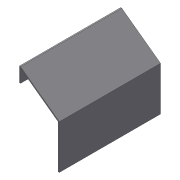
# Autodesk Inventor part: タイヤカバー
Saved by Autodesk Inventor 2020 (Build 240168000, 168)
## iProperties
Created: 2020-04-18
Part Number: タイヤカバー
Material: 一般
Document SubType Name: Modeling
Designer: highs
Density: 1 g/cm^3
Appearance: 既定
Author: highs
Autodesk Inventor part; units mm, degrees
ref_plane "YZ Plane" through (0, 0, 0) normal (1, 0, 0) x (0, 1, 0)
ref_plane "XZ Plane" through (0, 0, 0) normal (0, 1, 0) x (-1, 0, 0)
ref_plane "XY Plane" through (0, 0, 0) normal (0, 0, 1) x (1, 0, 0)
sketch "スケッチ1" plane through (0, 0, 0) normal (0, 0, 1) x (1, 0, 0)
  line L0 (0, 0) -> (0, 50)
  line L1 (0, 50) -> (4, 50)
  line L2 (4, 50) -> (138, -47.9694)
  line L3 (138, -47.9694) -> (138, -200)
  line L4 (138, -200) -> (134, -200)
  line L5 (134, -200) -> (134, -50)
  line L6 (134, -50) -> (4, 45.045)
  line L7 (0, 0) -> (4, 0)
  line L8 (4, 0) -> (4, 45.045)
  dimension "d0" = 4
  dimension "d1" = 4
  dimension "d2" = 4
  dimension "d3" = 50
  dimension "d4" = 250
  dimension "d5" = 134
  dimension "d6" = 4
  dimension "d8" = 150
  constraints: 18 end point, 3 parallel, 3 perpendicular, 1 horizontal, 1 vertical
  measures "d0" distance between parallel lines of L3 L5
  measures "d1" distance between parallel lines of L2 L6
  measures "d2" distance between parallel lines of L0 L8
  measures "d3" distance of L0.start L0.end
  measures "d4" distance between parallel lines of L4 L1
  measures "d5" distance between parallel lines of L5 L0
  measures "d6" distance of L0.end L1.end
  measures "d8" distance of L4.end L5.end
extrude "押し出し1" add sketch "スケッチ1" along normal blind 350
